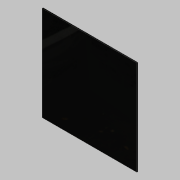
# Autodesk Inventor part: Base
Saved by Autodesk Inventor 2015 (Build 190159000, 159)
## iProperties
Created: 2015-03-03
Part Number: Base
Material: Generic
Document SubType Name: Modeling
Designer: Vukica
Density: 1 g/cm^3
Appearance: Glossy - Black
Author: Vukica
Autodesk Inventor part; units mm, degrees
ref_plane "YZ Plane" through (0, 0, 0) normal (1, 0, 0) x (0, 1, 0)
ref_plane "XZ Plane" through (0, 0, 0) normal (0, 1, 0) x (-1, 0, 0)
ref_plane "XY Plane" through (0, 0, 0) normal (0, 0, 1) x (1, 0, 0)
sketch "Sketch1" plane through (0, 0, 0) normal (0, 0, 1) x (1, 0, 0)
  line L0 (0, 0) -> (0, 9.6943) construction
  line L1 (0, 0) -> (12.344, 0) construction
  line L2 (-1219.2, 1219.2) -> (1219.2, 1219.2)
  line L3 (1219.2, 1219.2) -> (1219.2, -1219.2)
  line L4 (1219.2, -1219.2) -> (-1219.2, -1219.2)
  line L5 (-1219.2, -1219.2) -> (-1219.2, 1219.2)
  dimension "d0" = 2438.4
  dimension "d1" = 2438.4
  constraints: 12 end point, 3 horizontal, 2 parallel, 2 vertical, 1 perpendicular, 2 other
  measures "d0" distance of L3.end L4.end
  measures "d1" distance of L4.end L2.start
extrude "Extrusion1" add sketch "Sketch1" along normal blind 25.4
sketch "Sketch2" plane through (0, 0, 25.4) normal (0, 0, 1) x (1, 0, 0)
  line L0 (1524, -1079.5) -> (1524, 1079.5) projected
  line L1 (-1524, -1066.8) -> (1524, -1066.8) projected
  line L2 (-1524, 1079.5) -> (-1524, -1079.5) projected
  line L3 (1219.2, 1066.8) -> (-1219.2, 1066.8) projected
  line L4 (0, 76.2) -> (0, -1668.909) construction
  line L5 (1219.2, 1219.2) -> (-1219.2, 1219.2) projected
  line L6 (-635, 76.2) -> (-635, -1066.8)
  line L7 (635, -1066.8) -> (635, 76.2)
  arc A0 (635, 76.2) -> (-635, 76.2) centre (0, 76.2) ccw
  line L8 (635, -1066.8) -> (-635, -1066.8)
  point P0 (0, 0)
  point P1 (-1524, -1079.5)
  point P2 (0, -796.3545)
  dimension "d4" = 0
  dimension "d5" = 1270
  dimension "d6" = 1143
  constraints: 10 end point, 2 point on circle, 2 tangent, 1 centre point, 1 collinear, 1 horizontal, 1 midpoint, 1 parallel, 1 perpendicular, 1 vertical, 2 other
  measures "d4" distance from line of point (0, 0) L4
  measures "d5" distance between parallel lines of L6 L7
  measures "d6" distance of L6.start L6.end
extrude "Extrusion2" [suppressed]
sketch "Sketch3" plane through (0, 0, 25.4) normal (0, 0, 1) x (1, 0, 0)
  line L0 (1524, -381) -> (1143, -381) projected
  line L1 (-1524, -381) -> (-1143, -381) projected
  line L2 (1524, -1079.5) -> (1524, 1079.5) projected
  line L3 (-1524, 1079.5) -> (-1524, -1079.5) projected
  line L4 (1524, 1066.8) -> (-1524, 1066.8) projected
  arc A0 (658.9085, 247.4421) -> (-658.9085, 247.4421) centre (0, -760.7876) ccw
  line L5 (889, -762) -> (1143, -762) projected
  line L6 (889, -1066.8) -> (889, -762) projected
  line L7 (-1143, -762) -> (-889, -762) projected
  line L8 (889, -762) -> (889, -177.8)
  line L9 (-889, -762) -> (-889, -177.8)
  line L10 (-889, -1066.8) -> (-889, -762) projected
  line L11 (1143, -381) -> (1143, -762) projected
  line L12 (-1143, -762) -> (-1143, -381) projected
  arc A1 (889, -177.8) -> (658.9085, 247.4421) centre (381, -177.8) ccw
  arc A2 (-658.9085, 247.4421) -> (-889, -177.8) centre (-381, -177.8) ccw
  line L13 (-1219.2, -1219.2) -> (1219.2, -1219.2) projected
  arc A3 (635, 76.2) -> (-635, 76.2) centre (0, 76.2) ccw projected
  line L14 (914.4, 660.4) -> (939.8, 660.4) projected
  line L15 (668.6108, 660.4) -> (-668.6108, 660.4)
  arc A4 (1524, -381) -> (668.6108, 660.4) centre (0, -760.7876) ccw
  arc A5 (-668.6108, 660.4) -> (-1524, -381) centre (0, -760.7876) ccw
  point P0 (0, 0)
  point P1 (889, 51.8418)
  point P2 (-889, 51.8418)
  point P3 (635, -1066.8)
  dimension "d9" = 508
  dimension "d10" = 889
  constraints: 15 point on circle, 7 end point, 5 centre point, 4 tangent, 2 point on line, 2 vertical, 1 collinear, 1 equal radius, 1 horizontal, 3 other
  measures "d9" radius of A1
extrude "Extrusion3" [suppressed]
body "Solid1"
